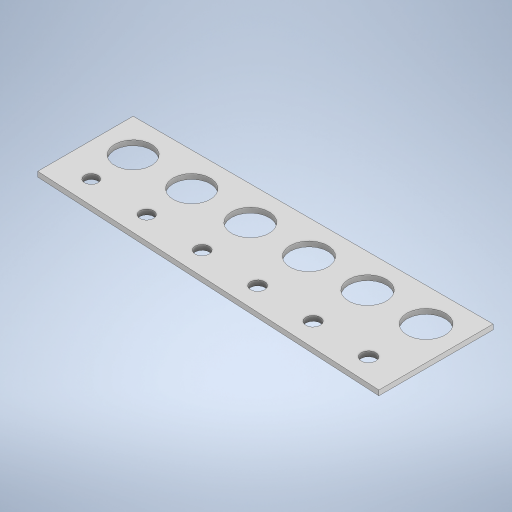
# Autodesk Inventor part: agujeros 8mm y 22mm
Saved by Autodesk Inventor 2024 (Build 280153000, 153)
## iProperties
Created: 2024-04-26
Part Number: agujeros 8mm y 22mm
Material: Generic
Document SubType Name: Modeling
Designer: compu
Density: 1 g/cm^3
Appearance: Default
Author: compu
Autodesk Inventor part; units mm, degrees
ref_plane "YZ Plane" through (0, 0, 0) normal (1, 0, 0) x (0, 1, 0)
ref_plane "XZ Plane" through (0, 0, 0) normal (0, 1, 0) x (-1, 0, 0)
ref_plane "XY Plane" through (0, 0, 0) normal (0, 0, 1) x (1, 0, 0)
sketch "Sketch1" plane through (0, 0, 0) normal (0, 1, 0) x (-1, 0, 0)
  line L0 (64.9523, 0) -> (-249.7137, 0) projected
  line L1 (0, -33.6475) -> (0, 61.8848) projected
  circle A0 centre (0, 0) radius 11
  circle A1 centre (-35, 0) radius 11.1
  circle A2 centre (-70, 0) radius 11.2
  circle A3 centre (-105, 0) radius 11.25
  circle A4 centre (-140, 0) radius 11.3
  circle A5 centre (-175, 0) radius 11.4
  line L2 (13.9808, 24.2673) -> (-204.7614, 35.7311) construction
  circle A6 centre (0, 25) radius 4
  circle A7 centre (-34.952, 26.8318) radius 4.1
  circle A8 centre (-69.9041, 28.6635) radius 4.2
  circle A9 centre (-104.8561, 30.4953) radius 4.25
  circle A10 centre (-139.8081, 32.327) radius 4.3
  circle A11 centre (-174.7602, 34.1588) radius 4.4
  line L3 (-195, -20) -> (-195, 48.2374)
  line L4 (20, 36.9697) -> (20, -20)
  line L5 (20, -20) -> (-195, -20)
  line L6 (20, 36.9697) -> (-195, 48.2374)
  dimension "d0" = 22
  dimension "d1" = 22.2
  dimension "d2" = 22.4
  dimension "d3" = 22.5
  dimension "d4" = 35
  dimension "d5" = 35
  dimension "d6" = 35
  dimension "d7" = 22.6
  dimension "d8" = 22.8
  dimension "d9" = 35
  dimension "d10" = 35
  dimension "d12" = 8
  dimension "d13" = 8.2
  dimension "d14" = 8.4
  dimension "d15" = 8.5
  dimension "d16" = 8.6
  dimension "d17" = 8.8
  dimension "d18" = 35
  dimension "d19" = 35
  dimension "d20" = 35
  dimension "d21" = 35
  dimension "d22" = 35
  dimension "d23" = 20
  dimension "d24" = 20
  dimension "d29" = 3
  dimension "d30" = 20
  dimension "d31" = 25
  dimension "d32" = 13
  constraints: 13 point on line, 12 centre point, 11 end point, 3 parallel, 1 coincident, 1 perpendicular
  measures "d0" diameter of A0
  measures "d1" diameter of A1
  measures "d2" diameter of A2
  measures "d3" diameter of A3
  measures "d4" distance of A1.centre A0.centre
  measures "d5" distance of A2.centre A1.centre
  measures "d6" distance of A3.centre A2.centre
  measures "d7" diameter of A4
  measures "d8" diameter of A5
  measures "d9" distance of A4.centre A3.centre
  measures "d10" distance of A5.centre A4.centre
  measures "d12" diameter of A6
  measures "d13" diameter of A7
  measures "d14" diameter of A8
  measures "d15" diameter of A9
  measures "d16" diameter of A10
  measures "d17" diameter of A11
  measures "d18" distance of A7.centre A6.centre
  measures "d19" distance of A8.centre A7.centre
  measures "d20" distance of A9.centre A8.centre
  measures "d21" distance of A10.centre A9.centre
  measures "d22" distance of A11.centre A10.centre
  measures "d23" distance from line of L4 point (0, 0)
  measures "d24" distance from line of L3 A5.centre
  measures "d29" angle of L6 L5
  measures "d30" distance from line of L5 point (0, 0)
  measures "d31" distance of A0.centre A6.centre
  measures "d32" distance between parallel lines of L6 L2
extrude "Extrusion1" add sketch "Sketch1" along normal blind 3 contours L4 L5 L1 A0 L0 | L0 A0 L1 A6 L6 L4 | A0 L0 A1 A2 A3 A4 A5 L3 L6 L1 A6 | L1 L5 L3 L0 A5 A4 A3 A2 A1 A0
body "Solid1"
